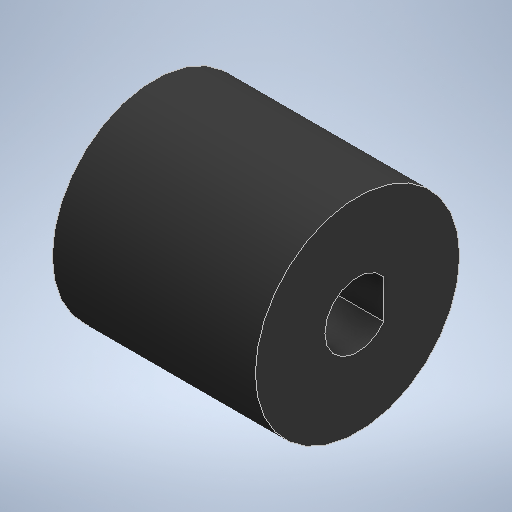
# Autodesk Inventor part: Roue test
Saved by Autodesk Inventor 2026.2 (Build 302298010, 298A)
## iProperties
Created: 2026-03-30
Part Number: Roue test
Material: Générique
Document SubType Name: Modeling
Designer: Genon
Density: 1 g/cm^3
Appearance: Caoutchouc - Noir
Author: Genon
Autodesk Inventor part; units mm, degrees
ref_plane "YZ Plane" through (0, 0, 0) normal (1, 0, 0) x (0, 1, 0)
ref_plane "XY Plane" through (0, 0, 0) normal (0, 0, 1) x (1, 0, 0)
sketch "Esquisse1" plane through (0, 0, 0) normal (0, 0, 1) x (1, 0, 0)
  line L0 (0, 0) -> (0, 38)
  line L1 (0, 38) -> (30, 38)
  line L2 (30, 38) -> (30, 35.5)
  line L3 (30, 35.5) -> (0, 35.5)
  line L4 (0, 0) -> (0, 10)
  line L5 (0, 10) -> (18, 10)
  line L6 (18, 10) -> (18, 0)
  line L7 (18, 0) -> (0, 0)
  line L8 (-6, 0) -> (36, 0) projected
  dimension "d0" = 38
  dimension "d1" = 30
  dimension "d2" = 2.5
  dimension "d3" = 10
  dimension "d4" = 18
  constraints: 16 end point, 6 perpendicular, 2 point on line, 1 vertical
  measures "d0" distance of L0.start L0.end
  measures "d1" distance of L0.end L1.end
  measures "d2" distance of L1.end L2.end
  measures "d3" distance of L0.start L4.end
  measures "d4" distance of L4.end L5.end
revolve "Révolution1" add sketch "Esquisse1" angle 360 about axis through (-10, 0, 0) along (1, 0, 0)
ref_plane "Plan de construction1" through (0, 10, 0) normal (0, 1, 0) x (-1, 0, 0)
sketch "Esquisse2" plane through (0, 10, 0) normal (0, 1, 0) x (-1, 0, 0)
  line L0 (0, 0) -> (0, 1)
  line L1 (0, 38) -> (0, -38) projected
  line L2 (0, 1) -> (-18, 1)
  line L3 (-18, 1) -> (-18, -1)
  line L4 (-18, -1) -> (0, -1)
  line L5 (0, 0) -> (0, -1)
  dimension "d7" = 1
  dimension "d8" = 18
  dimension "d9" = 2
  dimension "d10" = 90
  constraints: 10 end point, 3 perpendicular, 2 point on line, 1 collinear
  measures "d7" distance of L0.start L0.end
  measures "d8" distance of L0.end L2.end
  measures "d9" distance of L2.end L3.end
  measures "d10" angle of L3 L2
extrude "Extrusion1" add sketch "Esquisse2" along normal up to surface round surface about axis through (15, 0, 0) along (1, 0, 0) radius 35.5 far side no
sketch "Esquisse3" plane through (30, 0, 0) normal (1, 0, 0) x (0, 0, -1)
  circle A0 centre (0, 0) radius 38 projected
  circle A1 centre (0, 0) radius 38 projected
  line L0 (0, 38) -> (0, 40)
  line L1 (0, 40) -> (0.5, 40)
  line L2 (0.5, 40) -> (0.5, 37.9967)
  line L3 (0, 40) -> (-0.5, 40)
  line L4 (-0.5, 40) -> (-0.5, 37.9967)
  dimension "d13" = 2
  dimension "d14" = 0.5
  dimension "d15" = 0.5
  constraints: 10 end point, 3 perpendicular, 3 point on circle, 1 point on line, 1 vertical
  measures "d13" distance of L0.start L0.end
  measures "d14" distance of L0.end L1.end
  measures "d15" distance of L0.end L3.end
extrude "Extrusion2" add sketch "Esquisse3" against normal blind 30 contours A0 L0 L1 L2 | L4 L3 L0 A0
pattern_circular "Réseau circulaire1" count 10 over 360 about axis through (9, 0, 0) along (1, 0, 0) of "Extrusion1"
pattern_circular "Réseau circulaire2" count 40 over 360 about axis through (9, 0, 0) along (1, 0, 0) of "Extrusion2"
sketch "Esquisse4" plane through (0, 0, 0) normal (-1, 0, 0) x (0, 0, 1)
  circle A0 centre (0, 0) radius 2.25
  circle A1 centre (0, 0) radius 2.5
  line L0 (2.5, 0) -> (-1.816, 0)
  line L1 (-1.816, 0) -> (-1.816, 1.7182)
  line L2 (-1.816, 0) -> (-1.816, -1.7182)
  point P0 (-1.816, -1.3284)
  point P1 (-1.816, 1.3284)
  dimension "d24" = 4.5
  dimension "d25" = 5
  dimension "d26" = 4.316
  constraints: 6 end point, 3 point on circle, 2 centre point, 2 coincident, 1 horizontal, 1 perpendicular, 1 point on line
  measures "d24" diameter of A0
  measures "d25" diameter of A1
  measures "d26" distance of L0.start L0.end
extrude "Extrusion3" cut sketch "Esquisse4" against normal blind 25 contours L0 L1 A0 | A0 L2 L0
sketch "Esquisse7" plane through (0, 0, 0) normal (-1, 0, 0) x (0, 0, 1)
  circle A0 centre (0, 0) radius 2.5
  dimension "d30" = 5
  constraints: 1 centre point, 1 coincident
  measures "d30" diameter of A0
extrude "Extrusion4" cut sketch "Esquisse7" against normal blind 7
sketch "Esquisse8" plane through (0, 0, 0) normal (-1, 0, 0) x (0, 0, 1)
  circle A0 centre (0, 0) radius 2.5 projected
  circle A1 centre (0, 0) radius 35.5
  arc A2 (-1.816, -1.3284) -> (-1.816, 1.3284) centre (0, 0) ccw projected
  line L0 (-1.816, 1.3284) -> (-1.816, -1.3284) projected
  circle A3 centre (0, 0) radius 2.5 projected
  constraints: 1 centre point, 1 coincident
extrude "Extrusion5" cut sketch "Esquisse8" against normal blind 4 contours A0 | A1
sketch "Esquisse9" plane through (18, 0, 0) normal (1, 0, 0) x (0, 0, -1)
  circle A0 centre (0, 0) radius 2.5 projected
  circle A1 centre (0, 0) radius 7.0446
  circle A2 centre (0, 0) radius 44.6529
  constraints: 2 centre point, 2 coincident
extrude "Extrusion6" cut sketch "Esquisse9" along normal through all both and the other way through all contours A2
